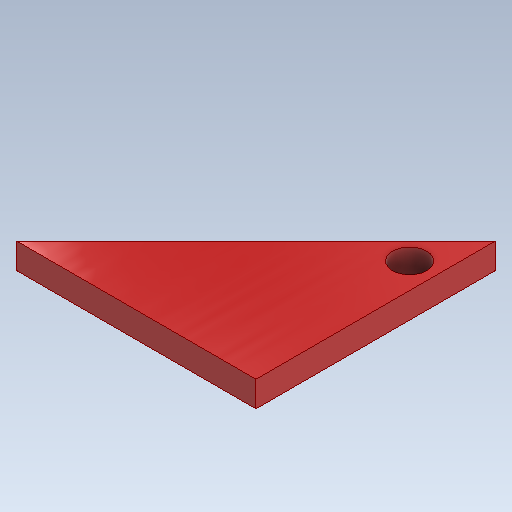
# Autodesk Inventor part: triangleSupportForMount
Saved by Autodesk Inventor 2021.1 (Build 251245010, 245A)
## iProperties
Created: 2020-11-06
Part Number: triangleSupportForMount
Material: PET Plastic
Document SubType Name: Modeling
Designer: robst
Density: 1.541 g/cm^3
Appearance: Red
Author: robst
Autodesk Inventor part; units mm, degrees
ref_plane "YZ Plane" through (0, 0, 0) normal (1, 0, 0) x (0, 1, 0)
ref_plane "XZ Plane" through (0, 0, 0) normal (0, 1, 0) x (-1, 0, 0)
ref_plane "XY Plane" through (0, 0, 0) normal (0, 0, 1) x (1, 0, 0)
sketch "Sketch1" plane through (0, 0, 0) normal (0, 1, 0) x (-1, 0, 0)
  line L0 (0, 0) -> (0, -177.8)
  line L1 (0, -177.8) -> (177.8, 0)
  line L2 (177.8, 0) -> (0, 0)
  dimension "d0" = 177.8
  dimension "d1" = 45
  constraints: 6 end point, 1 perpendicular, 1 vertical
  measures "d0" distance of L1.end L0.start
  measures "d1" angle of L1 L2
extrude "Extrusion1" add sketch "Sketch1" along normal mid plane 19.05
sketch "Sketch2" plane through (0, 9.525, 0) normal (0, 1, 0) x (1, 0, 0)
  line L0 (0, 0) -> (0, 177.8) projected
  line L1 (-23.8592, 127) -> (-22.225, 127) projected
  point P0 (-19.05, 133.35)
  dimension "d9" = 19.05
  dimension "d21" = 44.45
  measures "d9" distance from line of point (-19.05, 133.35) L0
  measures "d21" vertical distance of point (-19.05, 133.35) L0.end
hole "Hole1" at (-19.05, 9.525, -133.35) direction (0, -1, 0) diameter 25.4 end through all
equation "\"d5\" = wallWidth"
equation "\"wallWidth\" = 19.05"
body "Solid1"
